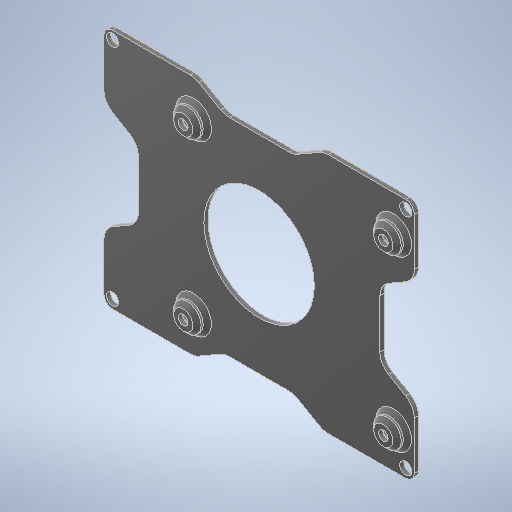
# Autodesk Inventor part: 3D_circuit-fix_raspberrypi
Saved by Autodesk Inventor 2025 (Build 290162000, 162)
## iProperties
Created: 2024-07-24
Part Number: 3D_circuit-fix_raspberrypi
Material: 一般
Document SubType Name: Modeling
Designer: 8326d
Density: 1 g/cm^3
Appearance: 滑らか - 黒
Author: 8326d
## iProperties of the stored document 3D_circuit-fix_raspberrypi_3D プリント.ipt
Created: 2024-08-08
Part Number: 3D_circuit-fix_raspberrypi_3D プリント
Material: 一般
Document SubType Name: Modeling
Designer: 8326d
Density: 1 g/cm^3
Appearance: 既定
Author: 8326d
Autodesk Inventor part; units mm, degrees
ref_plane "YZ Plane" through (0, 0, 0) normal (1, 0, 0) x (0, 1, 0)
ref_plane "XZ Plane" through (0, 0, 0) normal (0, 1, 0) x (-1, 0, 0)
ref_plane "XY Plane" through (0, 0, 0) normal (0, 0, 1) x (1, 0, 0)
sketch "スケッチ1" plane through (0, 0, 0) normal (0, 0, 1) x (1, 0, 0)
  line L0 (-45, -35) -> (45, -35)
  line L1 (45, -35) -> (45, 35)
  line L2 (45, 35) -> (-45, 35)
  line L3 (-45, 35) -> (-45, -35)
  line L4 (-45, -35) -> (45, 35) construction
  line L5 (45, -35) -> (-45, 35) construction
  point P0 (0, 0)
  dimension "d0" = 90
  dimension "d1" = 70
  constraints: 12 end point, 2 midpoint, 2 parallel, 1 horizontal, 1 perpendicular
  measures "d0" distance of L2.end L1.end
  measures "d1" distance of L1.end L0.end
extrude "押し出し1" add sketch "スケッチ1" along normal blind 1.2
sketch "スケッチ2" plane through (0, 0, 1.2) normal (0, 0, 1) x (1, 0, 0)
  line L0 (-42.5, -32.5) -> (42.5, -32.5) construction
  line L1 (42.5, -32.5) -> (42.5, 32.5) construction
  line L2 (42.5, 32.5) -> (-42.5, 32.5) construction
  line L3 (-42.5, 32.5) -> (-42.5, -32.5) construction
  line L4 (-42.5, -32.5) -> (42.5, 32.5) construction
  line L5 (42.5, -32.5) -> (-42.5, 32.5) construction
  point P0 (0, 0)
  dimension "d4" = 85
  dimension "d5" = 65
  constraints: 12 end point, 2 midpoint, 2 parallel, 1 horizontal, 1 perpendicular
  measures "d4" distance of L2.end L1.end
  measures "d5" distance of L1.end L0.end
hole "穴1" at (-42.5, 32.5, 1.2) at (-42.5, -32.5, 1.2) at (42.5, -32.5, 1.2) at (42.5, 32.5, 1.2) direction (0, 0, -1) diameter 3.5 end through all
sketch "スケッチ3" plane through (0, 0, 1.2) normal (0, 0, 1) x (1, 0, 0)
  circle A0 centre (-19, -24.5) radius 4
  circle A1 centre (-19, 24.5) radius 4
  circle A2 centre (39, 24.5) radius 4
  circle A3 centre (39, -24.5) radius 4
  point P0 (0, 0)
  dimension "d13" = 8
  dimension "d14" = 8
  dimension "d15" = 8
  dimension "d16" = 8
  dimension "d17" = 49
  dimension "d21" = 58
  dimension "d22" = 24.5
  dimension "d52" = 19
  constraints: 4 centre point, 2 horizontal alignment, 2 vertical alignment
  measures "d13" diameter of A0
  measures "d14" diameter of A1
  measures "d15" diameter of A2
  measures "d16" diameter of A3
  measures "d17" distance of A0.centre A1.centre
  measures "d21" distance of A3.centre A0.centre
  measures "d22" vertical distance of A0.centre point (0, 0)
  measures "d52" horizontal distance of point (0, 0) A1.centre
extrude "押し出し2" add sketch "スケッチ3" along normal blind 3
chamfer "面取り1" distance 1.2 angle 45 8 edges at (-23, -24.5, 4.2) (-23, 24.5, 4.2) (35, 24.5, 4.2) (35, -24.5, 4.2) (-23, 24.5, 1.2) (-23, -24.5, 1.2) (35, 24.5, 1.2) (35, -24.5, 1.2)
sketch "スケッチ4" plane through (-19, -24.5, 4.2) normal (0, 0, 1) x (1, 0, 0)
  circle A0 centre (0, 49) radius 2.8 projected
  circle A1 centre (0, 0) radius 2.8 projected
  circle A2 centre (58, 0) radius 2.8 projected
  circle A3 centre (58, 49) radius 2.8 projected
  point P0 (19, 24.5)
hole "穴2" at (-19, 24.5, 4.2) at (-19, -24.5, 4.2) at (39, -24.5, 4.2) at (39, 24.5, 4.2) direction (0, 0, -1) diameter 2.8 end through all
sketch "スケッチ5" plane through (0, 0, 0) normal (0, 0, -1) x (-1, 0, 0)
  circle A0 centre (19, -24.5) radius 1.4 projected
  circle A1 centre (19, 24.5) radius 1.4 projected
  circle A2 centre (-39, 24.5) radius 1.4 projected
  circle A3 centre (-39, -24.5) radius 1.4 projected
  line L0 (19, -27.4445) -> (16.45, -25.9722)
  line L1 (16.45, -25.9722) -> (16.45, -23.0278)
  line L2 (16.45, -23.0278) -> (19, -21.5555)
  line L3 (19, -21.5555) -> (21.55, -23.0278)
  line L4 (21.55, -23.0278) -> (21.55, -25.9722)
  line L5 (21.55, -25.9722) -> (19, -27.4445)
  line L6 (19, 21.5555) -> (16.45, 23.0278)
  line L7 (16.45, 23.0278) -> (16.45, 25.9722)
  line L8 (16.45, 25.9722) -> (19, 27.4445)
  line L9 (19, 27.4445) -> (21.55, 25.9722)
  line L10 (21.55, 25.9722) -> (21.55, 23.0278)
  line L11 (21.55, 23.0278) -> (19, 21.5555)
  circle A4 centre (-39, -24.5) radius 2.8 projected
  line L12 (-39, -27.4445) -> (-41.55, -25.9722)
  line L13 (-41.55, -25.9722) -> (-41.55, -23.0278)
  line L14 (-41.55, -23.0278) -> (-39, -21.5555)
  line L15 (-39, -21.5555) -> (-36.45, -23.0278)
  line L16 (-36.45, -23.0278) -> (-36.45, -25.9722)
  line L17 (-36.45, -25.9722) -> (-39, -27.4445)
  line L18 (-39, 21.5555) -> (-41.55, 23.0278)
  line L19 (-41.55, 23.0278) -> (-41.55, 25.9722)
  line L20 (-41.55, 25.9722) -> (-39, 27.4445)
  line L21 (-39, 27.4445) -> (-36.45, 25.9722)
  line L22 (-36.45, 25.9722) -> (-36.45, 23.0278)
  line L23 (-36.45, 23.0278) -> (-39, 21.5555)
  point P0 (0, 0)
  dimension "d36" = 5.1
  dimension "d37" = 5.1
  dimension "d38" = 5.1
  dimension "d39" = 5.1
  constraints: 48 end point, 4 coincident, 4 vertical alignment, 52 other
  measures "d36" distance between parallel lines of L3 L0
  measures "d37" distance between parallel lines of L9 L6
  measures "d38" distance between parallel lines of L12 L15
  measures "d39" distance between parallel lines of L21 L18
extrude "押し出し3" cut sketch "スケッチ5" against normal blind 3 contours A2 | A3 | L0 L1 L2 L3 L4 L5 | L6 L7 L8 L9 L10 L11 | L16 A4 L17 L12 L13 L14 L15 | A4 L15 L16 | L16 L17 A4 | A4 L14 L15 | L17 L12 A4 | A4 L13 L14 | L12 L13 A4 | L18 L19 L20 L21 L22 L23
sketch "スケッチ6" plane through (0, 0, 3) normal (0, 0, -1) x (-1, 0, 0)
  line L0 (21.55, -23.0278) -> (21.55, -25.9722) projected
  line L1 (19, -21.5555) -> (21.55, -23.0278) projected
  line L2 (16.45, -23.0278) -> (19, -21.5555) projected
  line L3 (16.45, -25.9722) -> (16.45, -23.0278) projected
  line L4 (19, -27.4445) -> (16.45, -25.9722) projected
  line L5 (21.55, -25.9722) -> (19, -27.4445) projected
  circle A0 centre (19, -24.5) radius 1.4 projected
  line L6 (21.55, 25.9722) -> (21.55, 23.0278) projected
  line L7 (19, 27.4445) -> (21.55, 25.9722) projected
  line L8 (16.45, 25.9722) -> (19, 27.4445) projected
  line L9 (16.45, 23.0278) -> (16.45, 25.9722) projected
  line L10 (19, 21.5555) -> (16.45, 23.0278) projected
  line L11 (21.55, 23.0278) -> (19, 21.5555) projected
  circle A1 centre (19, 24.5) radius 1.4 projected
  circle A2 centre (-39, 24.5) radius 1.4 projected
  line L12 (-36.45, 25.9722) -> (-36.45, 23.0278) projected
  line L13 (-39, 27.4445) -> (-36.45, 25.9722) projected
  line L14 (-41.55, 25.9722) -> (-39, 27.4445) projected
  line L15 (-41.55, 23.0278) -> (-41.55, 25.9722) projected
  line L16 (-39, 21.5555) -> (-41.55, 23.0278) projected
  line L17 (-36.45, 23.0278) -> (-39, 21.5555) projected
  circle A3 centre (-39, -24.5) radius 1.4 projected
  line L18 (-41.55, -25.9722) -> (-41.55, -23.0278) projected
  line L19 (-39, -27.4445) -> (-41.55, -25.9722) projected
  line L20 (-36.45, -25.9722) -> (-39, -27.4445) projected
  line L21 (-36.45, -23.0278) -> (-36.45, -25.9722) projected
  line L22 (-39, -21.5555) -> (-36.45, -23.0278) projected
  line L23 (-41.55, -23.0278) -> (-39, -21.5555) projected
  line L24 (21.55, -23.0278) -> (21.55, -25.9722) projected
  line L25 (21.55, -24.6443) -> (17.85, -26.7805)
  line L26 (17.6, -26.6362) -> (17.6, -22.3638)
  line L27 (17.85, -22.2195) -> (21.55, -24.3557)
  line L28 (21.55, -25.9722) -> (19, -27.4445) projected
  line L29 (19, -21.5555) -> (21.55, -23.0278) projected
  circle A4 centre (19, -24.5) radius 1.4 projected
  line L30 (16.45, 25.9722) -> (19, 27.4445) projected
  line L31 (17.6, 26.6362) -> (17.6, 22.3638)
  line L32 (17.85, 22.2195) -> (21.55, 24.3557)
  line L33 (21.55, 25.9722) -> (21.55, 23.0278) projected
  line L34 (21.55, 24.6443) -> (17.85, 26.7805)
  line L35 (21.55, 23.0278) -> (19, 21.5555) projected
  line L36 (19, 27.4445) -> (21.55, 25.9722) projected
  circle A5 centre (19, 24.5) radius 1.4 projected
  line L37 (-40.4, 22.3638) -> (-40.4, 26.6362)
  line L38 (-40.15, 26.7805) -> (-36.45, 24.6443)
  line L39 (-36.45, 25.9722) -> (-36.45, 23.0278) projected
  line L40 (-36.45, 24.3557) -> (-40.15, 22.2195)
  line L41 (-39, 27.4445) -> (-36.45, 25.9722) projected
  line L42 (-36.45, 23.0278) -> (-39, 21.5555) projected
  circle A6 centre (-39, 24.5) radius 1.4 projected
  line L43 (-36.45, -24.6443) -> (-40.15, -26.7805)
  line L44 (-40.4, -26.6362) -> (-40.4, -22.3638)
  line L45 (-40.15, -22.2195) -> (-36.45, -24.3557)
  line L46 (-36.45, -25.9722) -> (-39, -27.4445) projected
  line L47 (-39, -21.5555) -> (-36.45, -23.0278) projected
  circle A7 centre (-39, -24.5) radius 1.4 projected
  point P0 (0, 0)
  point P1 (21.55, 24.3557)
  point P2 (17.6, 26.6362)
  point P3 (21.55, -24.6443)
  constraints: 24 end point, 24 point on line, 12 tangent, 8 parallel, 4 vertical
extrude "押し出し4" add sketch "スケッチ6" along normal blind 0.2 contours L0 L27 L2 L1 | L0 L5 L4 L25 | L26 L4 L3 L2 | L6 L34 L8 L7 | L6 L11 L10 L32 | L31 L10 L9 L8 | L38 L14 L13 L12 | L40 L12 L17 L16 | L37 L16 L15 L14 | L45 L23 L22 L21 | L43 L21 L20 L19 | L44 L19 L18 L23
fillet "フィレット1" radius 2.5 4 edges at (-45, -35, 0.6) (-45, 35, 0.6) (45, -35, 0.6) (45, 35, 0.6)
sketch "スケッチ7" plane through (0, 0, 1.2) normal (0, 0, 1) x (1, 0, 0)
  line L0 (42.5, 35) -> (-42.5, 35) projected
  line L1 (-10, 35) -> (10, 35)
  line L2 (10, 35) -> (10, 30)
  line L3 (10, 30) -> (-10, 30)
  line L4 (-10, 30) -> (-10, 35)
  line L5 (-10, 30) -> (-18.6603, 35)
  line L6 (10, 30) -> (18.6603, 35)
  line L7 (45, -32.5) -> (45, 32.5) projected
  line L8 (45, 10) -> (35, 10)
  line L9 (35, 10) -> (35, -10)
  line L10 (35, -10) -> (45, -10)
  line L11 (45, -10) -> (45, 10)
  line L12 (35, 10) -> (45, 15.7735)
  line L13 (45, -32.5) -> (45, 32.5) projected
  line L14 (45, 0) -> (35, 0)
  point P0 (0, 0)
  point P1 (0, 35)
  dimension "d45" = 20
  dimension "d46" = 5
  dimension "d47" = 30
  dimension "d48" = 30
  dimension "d53" = 20
  dimension "d54" = 10
  constraints: 24 end point, 5 midpoint, 5 parallel, 5 point on line, 2 horizontal, 2 perpendicular
  measures "d45" distance of L2.end L3.end
  measures "d46" distance of L1.end L2.end
  measures "d47" angle of L0 L6
  measures "d48" angle of L0 L5
  measures "d53" distance of L8.end L9.end
  measures "d54" distance of L8.start L8.end
extrude "押し出し5" cut sketch "スケッチ7" against normal through all contours L6 L2 L0 | L2 L3 L4 L0 | L4 L5 L0 | L14 L9 L8 L7 | L8 L12 L7
mirror "ミラー1" about plane through (0, 0, 0) normal (0, 1, 0) of "押し出し5"
mirror "ミラー2" about plane through (0, 0, 0) normal (1, 0, 0) of "押し出し5", "ミラー1"
fillet "フィレット2" radius 5 16 edges at (-18.6603, -35, 0.6) (-10, -30, 0.6) (10, -30, 0.6) (18.6603, -35, 0.6) (10, 30, 0.6) (-10, 30, 0.6) (-18.6603, 35, 0.6) (18.6603, 35, 0.6) (-45, -15.7735, 0.6) (-35, -10, 0.6) (-35, 10, 0.6) (-45, 15.7735, 0.6) (45, -15.7735, 0.6) (35, -10, 0.6) (35, 10, 0.6) (45, 15.7735, 0.6)
sketch "スケッチ8" plane through (0, 0, 1.2) normal (0, 0, 1) x (1, 0, 0)
  circle A0 centre (0, 0) radius 16
  dimension "d55" = 32
  constraints: 1 centre point, 1 coincident
  measures "d55" diameter of A0
extrude "押し出し6" cut sketch "スケッチ8" against normal through all
equation "\"d22\" = 0.5 * d17"
equation "\"d37\" = d36"
equation "\"d38\" = d36"
equation "\"d39\" = d36"
equation "\"d48\" = d47"
